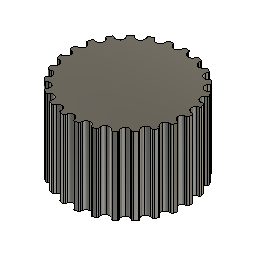
gear_25z (Autodesk Fusion 360 design; units mm, degrees)
Autodesk Fusion 360 part; units mm, degrees
sketch "Sketch1" plane through (0, 0, 0) normal (0, 0, 1) x (1, 0, 0) in component "gt2 pulley"
  circle A0 centre (0, 0) radius 7.9577 construction
  circle A1 centre (0, 0) radius 6.9537 construction
  line L0 (0, 0) -> (0, 7.9577) construction
  line L1 (0, 0) -> (0.9974, 7.895) construction
  line L2 (0, 0) -> (1.4111, 7.8316) construction
  circle A2 centre (0, 0) radius 7.7037 construction
  arc A3 (0.3664, 7.5547) -> (0.4111, 7.2847) centre (1.366, 7.5817) ccw
  circle A4 centre (0, 0) radius 7.5537 construction
  arc A5 (0.2207, 7.7006) -> (0, 7.7037) centre (0, 0) ccw
  arc A6 (0.3664, 7.5547) -> (0.2207, 7.7006) centre (0.2164, 7.5506) ccw
  arc A7 (0.4111, 7.2847) -> (0.8715, 6.8989) centre (0.9411, 7.4495) ccw
  arc A8 (0, 7.7037) -> (-0.2207, 7.7006) centre (0, 0) ccw
  arc A9 (-0.2207, 7.7006) -> (-0.3664, 7.5547) centre (-0.2164, 7.5506) ccw
  arc A10 (-0.4111, 7.2847) -> (-0.3664, 7.5547) centre (-1.366, 7.5817) ccw
  arc A11 (-0.8715, 6.8989) -> (-0.4111, 7.2847) centre (-0.9411, 7.4495) ccw
  arc A12 (0.8715, 6.8989) -> (-0.8715, 6.8989) centre (0, 0) ccw
  point P0 (1.366, 7.5817)
  point P1 (0, 7.7037)
  dimension "d18" = 15.9155
  dimension "d19" = 7.2
  dimension "d22" = 1.004
  dimension "d24" = 0.75
  dimension "d26" = 1
  dimension "d27" = 0.15
  dimension "d28" = 0.15
  dimension "d47" = 0.555
  dimension "d52" = 3.812
  constraint coincident A0.centre A1.centre
  constraint coincident A0 L0.end
  constraint vertical L0
  constraint coincident A0 L1.end
  constraint coincident A0 L2.end
  constraint concentric A1 A2
  constraint coincident A1 A7.end
  constraint coincident L1 A7.end
  constraint coincident A2 P0
  constraint coincident L2 P0
  constraint coincident P0 A3.centre
  constraint coincident A2 P1
  constraint coincident L0 P1
  constraint concentric A2 A4
  constraint coincident P1 A5.end
  constraint coincident A4 A6.centre
  constraint coincident A3.start A6.start
  constraint tangent A3 A6
  constraint tangent A3 A7
  constraint symmetric L0 A7.end A11.start
  constraint symmetric L0 A3.start A9.end
  constraint symmetric L0 A3.end A10.start
  constraint symmetric L0 A3 A10
  constraint symmetric L0 A5.start A8.end
  constraint symmetric L0 P1 A5.end
  constraint symmetric L0 A5 A8
  constraint symmetric L0 A6 A9
  constraint symmetric L0 A7 A11
  constraint coincident A1 A11.start
  constraint tangent A1 A7
  constraint coincident L1 A7.centre
  measures "d18" diameter of A0
  measures "d19" angle of L0 L1
  measures "d22" distance of A0 A1
  measures "d24" distance of A1 A2
  measures "d26" radius of A3
  measures "d27" distance of A2 A4
  measures "d28" radius of A6
  measures "d47" radius of A7
extrude "Extrude1" add sketch "Sketch1" along normal blind 10 makes body 1
pattern_circular "C-Pattern1" count 25 over 360 about axis through (0, 0, 1.75) along (0, 0, 1) of bodies 1 makes body 2 at (-1.0638, 6.8719, 3.3333) makes body 3 at (-3.4348, 6.0462, 6.6667) makes body 4 at (-4.8305, 5.0021, 6.6667) makes body 5 at (-5.9227, 3.6437, 6.6667) makes body 6 at (-6.7915, 1.4932, 6.6667) makes body 7 at (-6.8643, 1.1118, 3.3333) makes body 8 at (-6.9251, -0.6302, 3.3333) makes body 9 at (-6.25, -3.0483, 6.6667) makes body 10 at (-5.7649, -3.8885, 3.3333) makes body 11 at (-4.0084, -5.6822, 6.6667) makes body 12 at (-1.9167, -6.6844, 6.6667) makes body 13 at (-0.7751, -6.9104, 6.6667) makes body 14 at (1.5406, -6.7809, 6.6667) makes body 15 at (2.6499, -6.4291, 6.6667) makes body 16 at (4.1655, -5.5681, 6.6667) makes body 17 at (4.8998, -4.9342, 3.3333) makes body 18 at (6.3327, -2.8726, 6.6667) makes body 19 at (6.6708, -1.9633, 3.3333) makes body 20 at (6.9333, 0.5335, 6.6667) makes body 21 at (6.5828, 2.241, 6.6667) makes body 22 at (5.4796, 4.2812, 6.6667) makes body 23 at (5.2321, 4.5804, 3.3333) makes body 24 at (3.9286, 5.7376, 3.3333) makes body 25 at (1.6351, 6.7588, 6.6667)
sketch "Sketch2" plane through (0, 0, 10) normal (0, 0, 1) x (-1, 0, 0)
  arc A0 (-6.575, -3.7387) -> (-6.6201, -3.9399) centre (-6.4912, -3.8631) ccw
  arc A1 (-6.6201, -3.9399) -> (-6.3836, -4.3125) centre (0, 0) ccw
  arc A2 (-6.3836, -4.3125) -> (-6.1823, -4.3574) centre (-6.2592, -4.2286) ccw
  arc A3 (-5.9304, -4.2505) -> (-6.1823, -4.3574) centre (-5.6695, -5.2158) ccw
  arc A4 (-5.358, -4.4325) -> (-5.9304, -4.2505) centre (-5.7856, -4.7863) ccw
  arc A5 (-6.2919, -2.9608) -> (-5.358, -4.4325) centre (0, 0) ccw
  arc A6 (-6.371, -3.5562) -> (-6.2919, -2.9608) centre (-6.7941, -3.1971) ccw
  arc A7 (-6.575, -3.7387) -> (-6.371, -3.5562) centre (-7.1334, -2.9091) ccw
  circle A8 centre (0, 0) radius 6.9537
  constraint concentric A1 A8
extrude "Extrude2" add sketch "Sketch2" against normal blind 10 contours A5 A8 bodies 1 2 3 4 5 6 7 8 9 10 11 12 13 14 15 16 17 18 19 20 21 22 23 24 25
extrude "Extrude4" [suppressed] in component "gt2 pulley"
pattern_circular "C-Pattern7" [suppressed] in component "gt2 pulley"
extrude "Extrude3" [suppressed] in component "gt2 pulley"
pattern_circular "C-Pattern6" [suppressed] in component "gt2 pulley"
extrude "Extrude2'" [suppressed] in component "gt2 pulley"
pattern_circular "C-Pattern5" [suppressed] in component "gt2 pulley"
extrude "Extrude1'" [suppressed] in component "gt2 pulley"
pattern_circular "C-Pattern4" [suppressed] in component "gt2 pulley"
pattern_circular "C-Pattern3" [suppressed] in component "gt2 pulley"
pattern_circular "C-Pattern2" [suppressed] in component "gt2 pulley"
pattern_circular "C-Pattern1'" [suppressed] in component "gt2 pulley"
copy_body "Body->Comp1" [suppressed] in component "Component"
copy_body "Body->Comp2" [suppressed] in component "Component'"
copy_body "Body->Comp3" [suppressed] in component "Component''"
copy_body "Body->Comp4" [suppressed] in component "Component'''"
copy_body "Body->Comp5" [suppressed] in component "Component''''"
copy_body "Body->Comp6" [suppressed] in component "Component'''''"
copy_body "Body->Comp7" [suppressed] in component "Component''''''"
copy_body "Body->Comp8" [suppressed] in component "Component'''''''"
copy_body "Body->Comp9" [suppressed] in component "Component''''''''"
copy_body "Body->Comp10" [suppressed] in component "Component'''''''''"
copy_body "Body->Comp11" [suppressed] in component "Component''''''''''"
copy_body "Body->Comp12" [suppressed] in component "Component'''''''''''"
copy_body "Body->Comp13" [suppressed] in component "Component''''''''''''"
copy_body "Body->Comp14" [suppressed] in component "Component'''''''''''''"
copy_body "Body->Comp15" [suppressed] in component "Component''''''''''''''"
copy_body "Body->Comp16" [suppressed] in component "Component'''''''''''''''"
copy_body "Body->Comp17" [suppressed] in component "Component''''''''''''''''"
copy_body "Body->Comp18" [suppressed] in component "Component'''''''''''''''''"
copy_body "Body->Comp19" [suppressed] in component "Component''''''''''''''''''"
copy_body "Body->Comp20" [suppressed] in component "Component'''''''''''''''''''"
component "gt2 pulley" placed x (1, 0, 0) y (0, 1, 0) z (0, 0, 1) at (0, 0, 0)
equation "NumTeeth = 25" comment "min 20"
equation "ToothPitch = 2 mm"
equation "PullyDia = NumTeeth * ToothPitch / PI"
equation "ToothAng = ( ( 360 / NumTeeth ) * 1 deg )"
equation "TransOffsetAngle = ToothAng * 0.2"
equation "Sholulder_Radius = 0.15 mm"
equation "Root_Radius = 0.555 mm"
equation "TransRadius = 1 mm"
equation "ToolHeight = 0.75 mm"
equation "PLD = 0.254 mm"
equation "d18 = PullyDia"
equation "d19 = ToothAng / 2"
equation "d22 = PLD + ToolHeight"
equation "d24 = ToolHeight"
equation "d26 = TransRadius"
equation "d27 = Sholulder_Radius"
equation "d31 = NumTeeth"
equation "d33 = NumTeeth"
equation "d35 = NumTeeth"
equation "d37 = NumTeeth"
equation "d41 = NumTeeth"
equation "d45 = NumTeeth"
equation "d47 = Root_Radius"
equation "d50 = NumTeeth"
